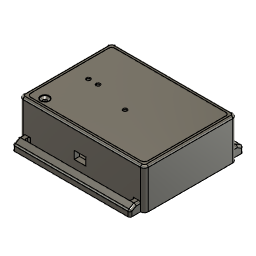
V5.0 Open-Source (Autodesk Fusion 360 design; units mm, degrees)
Autodesk Fusion 360 part; units mm, degrees
sketch "Top" plane through (0, 0, 0) normal (0, 1, 0) x (1, 0, 0)
  line L0 (35, -26.2) -> (48.95, -26.2) construction
  arc A0 (63, -48) -> (65, -46) centre (63, -46) ccw
  line L1 (63, -44) -> (63, -2)
  line L2 (38.05, -45.263) -> (25.05, -45.263)
  circle A1 centre (35, -26.2) radius 1.75
  line L3 (61.65, -14) -> (63, -14)
  line L4 (50.95, -35.25) -> (33, -35.25)
  line L5 (65, -2) -> (0, -2) construction
  circle A2 centre (35, -26.2) radius 1.4
  line L6 (39.475, -32.2956) -> (39.475, -27.2956)
  circle A3 centre (48.95, -26.2) radius 1.75
  line L7 (41.975, -26.2) -> (41.975, -27.2956) construction
  circle A4 centre (59.92, -22.92) radius 0.9 construction
  line L8 (58.127, -46) -> (58.127, -20.5)
  line L9 (25.05, -38.863) -> (38.05, -38.863) construction
  line L10 (30.3, -22) -> (33, -22)
  line L11 (2, 0) -> (63, 0)
  line L12 (2, -48) -> (63, -48)
  line L13 (39.55, -38.863) -> (39.55, -46) construction
  line L14 (3.35, -14) -> (2, -14)
  line L15 (29.5, -20.5) -> (29.5, -46) construction
  line L16 (2, -22) -> (30.3, -22) construction
  line L17 (63, -2) -> (2, -2)
  line L18 (63, -48) -> (63, 0) construction
  line L19 (61, -46) -> (4, -46)
  circle A5 centre (59.92, -43.58) radius 0.9 construction
  line L20 (25.05, -45.263) -> (25.05, -46)
  line L21 (50.95, -22) -> (58.127, -22)
  line L22 (38.05, -45.263) -> (38.05, -46)
  line L23 (38.05, -38.863) -> (39.55, -38.863) construction
  line L24 (33, -35.25) -> (33, -22)
  arc A6 (61, -46) -> (63, -44) centre (61, -44) ccw
  line L25 (2, -22) -> (0, -22) construction
  line L26 (2, -39.4) -> (30.3, -39.4)
  line L27 (30.3, -22) -> (30.3, -39.4)
  line L28 (2, -35.05) -> (25.085, -35.05)
  line L29 (39.475, -27.2956) -> (44.475, -27.2956)
  line L30 (44.475, -32.2956) -> (39.475, -32.2956)
  line L31 (2, -26.35) -> (25.085, -26.35)
  arc A7 (2, -44) -> (4, -46) centre (4, -44) ccw
  line L32 (33, -22) -> (50.95, -22)
  line L33 (65, -2) -> (65, -46)
  line L34 (0, -46) -> (0, -2)
  arc A8 (0, -46) -> (2, -48) centre (2, -46) ccw
  line L35 (38.05, -38.863) -> (38.05, -45.263) construction
  line L36 (25.085, -26.35) -> (25.085, -35.05)
  line L37 (6.88, -36.96) -> (6.88, -22) construction
  line L38 (25.05, -45.263) -> (25.05, -38.863) construction
  line L39 (23.55, -39.4) -> (23.55, -46)
  line L40 (0, -36.96) -> (6.88, -36.96) construction
  line L41 (2, -2) -> (2, -44)
  line L42 (8.127, -20.5) -> (8.127, -22)
  arc A9 (2, 0) -> (0, -2) centre (2, -2) ccw
  circle A10 centre (48.95, -26.2) radius 1.4
  line L43 (50.95, -22) -> (50.95, -35.25)
  line L44 (30.3, -39.4) -> (39.55, -39.4)
  arc A11 (65, -2) -> (63, 0) centre (63, -2) ccw
  line L45 (44.475, -27.2956) -> (44.475, -32.2956)
  line L46 (61.65, -17.5) -> (3.35, -17.5)
  line L47 (61.65, -14) -> (61.65, -2)
  line L48 (61.65, -17.5) -> (61.65, -14)
  line L49 (3.35, -14) -> (3.35, -2)
  line L50 (3.35, -17.5) -> (3.35, -14)
  line L51 (63, -19) -> (8.127, -19)
  line L52 (0, 0) -> (2, 0) construction
  line L53 (0, 0) -> (0, -2) construction
  line L54 (8.127, -20.5) -> (8.127, -19)
  circle A12 centre (8, -42.7) radius 2
  circle A13 centre (8, -42.7) radius 1
  line L55 (10.5, -46) -> (10.5, -39.4)
  line L56 (8.127, -22) -> (30.3, -22)
  line L57 (25.05, -39.4) -> (25.05, -45.263)
  line L58 (39.55, -39.4) -> (39.55, -46)
  line L59 (38.05, -39.4) -> (38.05, -45.263)
  line L60 (29.5, -20.5) -> (29.5, -22)
  line L61 (8.127, -20.5) -> (63, -20.5)
  line L62 (29.5, -22.6364) -> (36.034, -22.6364) construction
  line L63 (36.034, -22.6364) -> (36.9763, -20.5) construction
  line L64 (5.5, -39.4) -> (5.5, -46)
  line L65 (5.5, -45.2) -> (10.5, -45.2)
  line L66 (10.5, -40.2) -> (5.5, -40.2)
  line L67 (36.2744, -22) -> (36.936, -20.5)
  point P0 (0, -48)
  point P1 (65, 0)
  dimension "d1" = 65
  dimension "d2" = 48
  dimension "d3" = 2
  dimension "d9" = 2
  dimension "d10" = 2
  dimension "d11" = 33.5
  dimension "d12" = 4.873
  dimension "d14" = 13.25
  dimension "d15" = 17.95
  dimension "d16" = 3.5
  dimension "d17" = 2
  dimension "d18" = 28.3
  dimension "d19" = 28.3
  dimension "d20" = 17.4
  dimension "d22" = 6.88
  dimension "d23" = 14.96
  dimension "d24" = 2
  dimension "d26" = 6.4
  dimension "d27" = 13
  dimension "d28" = 0.737
  dimension "d29" = 23.05
  dimension "d30" = 1.8
  dimension "d31" = 1.8
  dimension "d32" = 2.42
  dimension "d33" = 3.08
  dimension "d34" = 3.08
  dimension "d36" = 3.5
  dimension "d37" = 3.5
  dimension "d38" = 2
  dimension "d39" = 2
  dimension "d40" = 4.2
  dimension "d41" = 4.2
  dimension "d42" = 90
  dimension "d44" = 5
  dimension "d45" = 5
  dimension "d46" = 90
  dimension "d47" = 2.8
  dimension "d48" = 2.8
  dimension "d49" = 1.5
  dimension "d50" = 1.5
  dimension "d51" = 4.35
  dimension "d129" = 2
  dimension "d133" = 2.9544
  dimension "d134" = 4.35
  dimension "d135" = 5.215
  dimension "d139" = 0.537
  dimension "d140" = 1.35
  dimension "d141" = 1.35
  dimension "d142" = 15.5
  dimension "d143" = 1.5
  dimension "d146" = 2
  dimension "d147" = 50
  dimension "d148" = 12
  dimension "d149" = 12
  dimension "d163" = 4
  dimension "d164" = 3.3
  dimension "d165" = 6
  dimension "d166" = 2
  dimension "d167" = 2.5
  dimension "d208" = 25.5
  dimension "d266" = 6.534
  dimension "d267" = 113.8
  dimension "d268" = 2.335
  dimension "d397" = 2.5
  dimension "d398" = 2.5
  dimension "d399" = 2.5
  dimension "d421" = 7.436
  constraint vertical L33
  constraint coincident L52.start L53.start
  constraint coincident L5.start L33
  constraint coincident L5.end L34
  constraint perpendicular L5 L34
  constraint coincident L1.end L18
  constraint coincident L1.end L5
  constraint coincident L17.end L5
  constraint coincident L3.end L18
  constraint perpendicular L3 L18
  constraint perpendicular L12 L33
  constraint coincident A0.start L12
  constraint perpendicular L11 L33
  constraint coincident L18.end L11
  constraint coincident L52.start L34
  constraint coincident L52.start L11
  constraint tangent L34 A9
  constraint tangent L11 A9
  constraint coincident P0 L34
  constraint coincident P0 L12
  constraint tangent L34 A8
  constraint tangent L12 A8
  constraint equal A8 A9
  constraint tangent A0 L33
  constraint tangent A0 L12
  constraint equal A0 A9
  constraint coincident P1 L33
  constraint coincident P1 L11
  constraint tangent L33 A11
  constraint tangent L11 A11
  constraint equal A9 A11
  constraint coincident L15.end L19
  constraint perpendicular L15 L19
  constraint coincident L8.start L19
  constraint horizontal L32
  constraint vertical L43
  constraint horizontal L4
  constraint vertical L24
  constraint tangent A7 L41
  constraint tangent L19 A7
  constraint tangent L19 A6
  constraint tangent L1 A6
  constraint equal A6 A7
  constraint coincident L26.start L41
  constraint perpendicular L26 L41
  constraint coincident L40.start L34
  constraint perpendicular L34 L40
  constraint coincident L37.end L16
  constraint perpendicular L16 L37
  constraint coincident L25.end L34
  constraint perpendicular L25 L34
  constraint horizontal L9
  constraint vertical L35
  constraint horizontal L2
  constraint vertical L38
  constraint coincident L42.end L16
  constraint perpendicular L16 L42
  constraint parallel L10 L32
  constraint coincident L21.end L8
  constraint perpendicular L8 L21
  constraint horizontal L29
  constraint vertical L45
  constraint horizontal L30
  constraint vertical L6
  constraint coincident L0.start A1.centre
  constraint coincident L0.end A3.centre
  constraint midpoint L7.start L0
  constraint midpoint L7.end L29
  constraint concentric A1 A2
  constraint concentric A3 A10
  constraint coincident L22.end L19
  constraint perpendicular L19 L22
  constraint coincident L20.end L19
  constraint perpendicular L19 L20
  constraint perpendicular L20 L23
  constraint coincident L13.end L19
  constraint perpendicular L13 L19
  constraint coincident L39.start L26
  constraint coincident L39.end L19
  constraint perpendicular L19 L39
  constraint coincident L44.end L13
  constraint perpendicular L13 L44
  constraint coincident L14.end L41
  constraint coincident L31.start L41
  constraint perpendicular L31 L41
  constraint coincident L28.start L41
  constraint perpendicular L28 L37
  constraint perpendicular L28 L36
  constraint coincident L17 L47.end
  constraint perpendicular L3 L47
  constraint perpendicular L3 L48
  constraint coincident L17 L49.end
  constraint perpendicular L14 L49
  constraint perpendicular L14 L50
  constraint coincident L1 L51.start
  constraint perpendicular L41 L51
  constraint tangent A9 L52
  constraint concentric A12 A13
  constraint coincident L19 L55.start
  constraint coincident L26 L55.end
  constraint perpendicular L26 L55
  constraint coincident L26 L57.start
  constraint coincident L38 L57.start
  constraint coincident L35 L59.start
  constraint coincident L44 L59.start
  constraint coincident L16 L60.end
  constraint coincident L1 L61.end
  constraint coincident L8.end L61
  constraint coincident L15.start L61
  constraint perpendicular L1 L61
  constraint perpendicular L54 L61
  constraint perpendicular L60 L61
  constraint coincident L15 L62.start
  constraint perpendicular L24 L62
  constraint coincident L61 L63.end
  constraint coincident L26 L64.start
  constraint coincident L19 L64.end
  constraint perpendicular L19 L64
  constraint coincident L64 L65.start
  constraint coincident L55 L65.end
  constraint perpendicular L55 L65
  constraint coincident L55 L66.start
  constraint coincident L64 L66.end
  constraint perpendicular L64 L66
  constraint coincident L32 L67.start
  constraint coincident L61 L67.end
  constraint parallel L63 L67
  measures "d1" distance of P1 L52.start
  measures "d2" distance of P0 L52.start
  measures "d3" distance of L18 L33
  measures "d9" radius of A9
  measures "d10" distance of L11 L17
  measures "d11" distance of L1 L15
  measures "d12" distance of L1 L8
  measures "d14" distance of L4 L32
  measures "d15" distance of L24 L43
  measures "d16" distance of L15 L24
  measures "d17" radius of A7
  measures "d18" distance of L26.start L26.end
  measures "d19" distance of L10.start L16.start
  measures "d20" distance of L16 L26
  measures "d22" distance of L37.start L40.start
  measures "d23" distance of L37.start L37.end
  measures "d24" distance of L34 L41
  measures "d26" distance of L2.end L9.start
  measures "d27" distance of L35 L38
  measures "d28" distance of L2 L19
  measures "d29" distance of L38 L41
  measures "d30" diameter of A5
  measures "d31" diameter of A4
  measures "d32" distance of A5.centre L19
  measures "d33" distance of A5.centre L1
  measures "d34" distance of A4.centre L18
  measures "d36" diameter of A1
  measures "d37" diameter of A3
  measures "d38" distance of L0.end L43
  measures "d39" distance of L0.start L24
  measures "d40" distance of L0.start L32
  measures "d41" distance of L0.end L32
  measures "d42" angle of L10 L27
  measures "d44" distance of L30.start L29.end
  measures "d45" distance of L6 L45
  measures "d46" angle of L0 L7
  measures "d47" diameter of A2
  measures "d48" diameter of A10
  measures "d49" distance of L9.end L13.start
  measures "d50" distance of L38 L39
  measures "d51" distance of L26 L28
  measures "d129" distance of L12 L19
  measures "d133" distance of L4 L30
  measures "d134" distance of L16 L31
  measures "d135" distance of L27 L36
  measures "d139" distance of L9 L26
  measures "d140" distance of L1 L47
  measures "d141" distance of L41 L49
  measures "d142" distance of L17 L46
  measures "d143" distance of L46 L51
  measures "d146" distance of L11.start L52.start
  measures "d147" distance of L8 L42
  measures "d148" distance of L14 L17
  measures "d149" distance of L3 L17
  measures "d163" diameter of A12
  measures "d164" distance of L19 A12.centre
  measures "d165" distance of L41 A12.centre
  measures "d166" diameter of A13
  measures "d167" distance of A12.centre L55
  measures "d208" distance of L19 L61
  measures "d266" distance of L62.start L62.end
  measures "d267" angle of L61 L63
  measures "d268" distance of L62.end L63.end
  measures "d397" distance of A12.centre L64
  measures "d398" distance of A12.centre L66
  measures "d399" distance of A12.centre L65
  measures "d421" distance of L15 L67.end
sketch "TP4056+JST" plane through (0, 0, 0) normal (1, 0, 0) x (0, 0, -1)
  line L0 (-22, 4.5) -> (-39.4, 4.5) construction
  line L1 (-26.4, 5.78) -> (-26.4, 5.86)
  arc A0 (-33.87, 8.205) -> (-35.87, 6.205) centre (-33.87, 6.205) ccw
  line L2 (-25.53, 5.435) -> (-25.53, 6.205)
  arc A1 (-35.87, 5.435) -> (-33.87, 3.435) centre (-33.87, 5.435) ccw
  arc A2 (-35, 5.78) -> (-33.65, 4.43) centre (-33.65, 5.78) ccw
  line L3 (-22, 3) -> (-22, 4.5) construction
  line L4 (-27.75, 7.21) -> (-33.65, 7.21)
  arc A3 (-27.75, 4.43) -> (-26.4, 5.78) centre (-27.75, 5.78) ccw
  arc A4 (-27.53, 3.435) -> (-25.53, 5.435) centre (-27.53, 5.435) ccw
  line L5 (-39.4, 4.5) -> (-39.4, 3) construction
  arc A5 (-25.53, 6.205) -> (-27.53, 8.205) centre (-27.53, 6.205) ccw
  line L6 (-33.87, 3.435) -> (-27.53, 3.435)
  line L7 (-35.87, 5.435) -> (-37.96, 5.435)
  line L8 (-37.96, 5.435) -> (-37.96, 8.435)
  line L9 (-35, 5.86) -> (-35, 5.78)
  line L10 (-33.65, 4.43) -> (-27.75, 4.43)
  line L11 (-30.7, 3) -> (-30.7, 7.21) construction
  line L12 (-25.53, 5.435) -> (-23.44, 5.435)
  line L13 (-27.53, 8.205) -> (-33.87, 8.205)
  arc A6 (-33.65, 7.21) -> (-35, 5.86) centre (-33.65, 5.86) ccw
  line L14 (-35.87, 6.205) -> (-35.87, 5.435)
  arc A7 (-26.4, 5.86) -> (-27.75, 7.21) centre (-27.75, 5.86) ccw
  line L15 (-23.44, 5.435) -> (-23.44, 8.435)
  line L16 (-39.4, 3) -> (-22, 3) construction
  line L17 (0, 0) -> (-48, 0)
  line L18 (-48, 0) -> (-48, 21)
  line L19 (-48, 21) -> (0, 21)
  line L20 (0, 21) -> (0, 0)
  line L21 (-25.44, 10.435) -> (-35.96, 10.435)
  line L22 (-44, 6) -> (-44, 9)
  line L23 (-43, 5) -> (-40, 5)
  line L24 (-39, 6) -> (-39, 9)
  line L25 (-40, 10) -> (-43, 10)
  arc A8 (-39, 9) -> (-40, 10) centre (-40, 9) ccw
  arc A9 (-43, 10) -> (-44, 9) centre (-43, 9) ccw
  arc A10 (-44, 6) -> (-43, 5) centre (-43, 6) ccw
  arc A11 (-40, 5) -> (-39, 6) centre (-40, 6) ccw
  line L26 (-37.96, 5.435) -> (-37.96, 3)
  line L27 (-23.44, 5.435) -> (-23.44, 3)
  line L28 (-25.53, 5.435) -> (-26.4448, 5.435)
  line L29 (-35.87, 5.435) -> (-34.9552, 5.435)
  line L30 (-23.44, 3) -> (-23.44, 1.5)
  line L31 (-23.44, 1.5) -> (-37.96, 1.5)
  line L32 (-37.96, 1.5) -> (-37.96, 3)
  arc A12 (-23.44, 8.435) -> (-25.44, 10.435) centre (-25.44, 8.435) ccw
  arc A13 (-35.96, 10.435) -> (-37.96, 8.435) centre (-35.96, 8.435) ccw
  point P0 (-26.4, 7.21)
  point P1 (-26.4, 4.43)
  point P2 (-35, 7.21)
  point P3 (-35.87, 8.205)
  point P4 (-25.53, 8.205)
  point P5 (-25.53, 3.435)
  point P6 (-23.44, 10.435)
  point P7 (-44, 5)
  dimension "d58" = 1.5
  dimension "d59" = 17.4
  dimension "d62" = 8.6
  dimension "d63" = 2.78
  dimension "d64" = 1.43
  dimension "d65" = 90
  dimension "d66" = 1.35
  dimension "d67" = 10.34
  dimension "d68" = 4.77
  dimension "d69" = 5.17
  dimension "d70" = 0.995
  dimension "d71" = 2
  dimension "d76" = 2.09
  dimension "d150" = 48
  dimension "d151" = 21
  dimension "d153" = 3.435
  dimension "d155" = 0.87
  dimension "d206" = 30.7
  dimension "d330" = 2.09
  dimension "d341" = 4
  dimension "d342" = 5
  dimension "d343" = 5
  dimension "d344" = 5
  dimension "d345" = 1
  dimension "d422" = 1.5
  dimension "d430" = 2
  dimension "d431" = 5
  constraint horizontal L0
  constraint vertical L5
  constraint horizontal L16
  constraint vertical L3
  constraint horizontal L4
  constraint vertical L9
  constraint horizontal L10
  constraint vertical L1
  constraint midpoint L11.start L16
  constraint coincident L11.end L4
  constraint coincident P0 L4
  constraint coincident P0 L1
  constraint tangent L4 A7
  constraint tangent L1 A7
  constraint coincident P2 L4
  constraint coincident P2 L9
  constraint tangent L4 A6
  constraint tangent L9 A6
  constraint equal A6 A7
  constraint tangent A2 L9
  constraint tangent A2 L10
  constraint equal A2 A7
  constraint coincident P1 L10
  constraint coincident P1 L1
  constraint tangent A3 L10
  constraint tangent L1 A3
  constraint equal A3 A7
  constraint horizontal L13
  constraint vertical L14
  constraint horizontal L6
  constraint vertical L2
  constraint coincident P4 L13
  constraint coincident P4 L2
  constraint tangent A5 L13
  constraint tangent L2 A5
  constraint coincident P3 L13
  constraint coincident P3 L14
  constraint tangent A0 L13
  constraint tangent A0 L14
  constraint equal A0 A5
  constraint tangent A1 L14
  constraint tangent A1 L6
  constraint equal A1 A5
  constraint coincident P5 L6
  constraint coincident P5 L2
  constraint tangent A4 L6
  constraint tangent L2 A4
  constraint equal A4 A5
  constraint perpendicular L2 L12
  constraint horizontal L17
  constraint vertical L18
  constraint horizontal L19
  constraint vertical L20
  constraint coincident L17.start L20.end
  constraint perpendicular L7 L8
  constraint horizontal L21
  constraint perpendicular L15 L21
  constraint vertical L22
  constraint perpendicular L22 L23
  constraint perpendicular L23 L24
  constraint perpendicular L24 L25
  constraint tangent L24 A8
  constraint tangent L25 A8
  constraint tangent L22 A9
  constraint tangent L25 A9
  constraint equal A8 A9
  constraint coincident P7 L22
  constraint coincident P7 L23
  constraint tangent L22 A10
  constraint tangent L23 A10
  constraint equal A8 A10
  constraint tangent L23 A11
  constraint tangent L24 A11
  constraint equal A8 A11
  constraint perpendicular L16 L26
  constraint coincident L16 L27.end
  constraint perpendicular L16 L27
  constraint coincident A3 L28.end
  constraint perpendicular L2 L28
  constraint coincident A2 L29.end
  constraint perpendicular L14 L29
  constraint perpendicular L16 L30
  constraint perpendicular L26 L31
  constraint perpendicular L16 L32
  constraint coincident P6 L15
  constraint tangent L21 A12
  constraint tangent L15 A12
  constraint tangent L8 A13
  constraint tangent L21 A13
  constraint equal A12 A13
  measures "d58" distance of L0 L16
  measures "d59" distance of L5.end L3.start
  measures "d62" distance of P0 P2
  measures "d63" distance of P0 P1
  measures "d64" distance of L10 L16
  measures "d65" angle of L11 L16
  measures "d66" radius of A7
  measures "d67" distance of P3 P4
  measures "d68" distance of P4 P5
  measures "d69" distance of L2 L11
  measures "d70" distance of L4 L13
  measures "d71" radius of A5
  measures "d76" distance of L2.start L12.end
  measures "d150" distance of L17.start L17.end
  measures "d151" distance of L17.start L19.end
  measures "d153" distance of L6 L17
  measures "d155" distance of L1 L2
  measures "d206" distance of L11 L20
  measures "d330" distance of L8 L14
  measures "d341" distance of L18 L22
  measures "d342" distance of L17 P7
  measures "d343" distance of L22 L24
  measures "d344" distance of L23 L25
  measures "d345" radius of A8
  measures "d422" distance of L17 L31
  measures "d430" radius of A12
  measures "d431" distance of L7 L21
ref_plane "WorkPlane2" through (0, 19, 0) normal (0, 1, 0) x (0, 0, 1)
sketch "Lid" plane through (0, 19, 0) normal (0, 1, 0) x (1, 0, 0)
  line L0 (0, 0) -> (65, 0) construction
  line L1 (65, 0) -> (65, -48) construction
  line L2 (65, -48) -> (0, -48) construction
  line L3 (0, -48) -> (0, 0) construction
  line L4 (62.95, -3.55) -> (62.95, -43.95)
  line L5 (60.95, -45.95) -> (4.05, -45.95)
  line L6 (2.05, -43.95) -> (2.05, -3.55)
  line L7 (3.55, -2.05) -> (61.45, -2.05)
  arc A0 (2.05, -43.95) -> (4.05, -45.95) centre (4.05, -43.95) ccw
  arc A1 (60.95, -45.95) -> (62.95, -43.95) centre (60.95, -43.95) ccw
  line L8 (2.05, -39.4) -> (30.35, -39.4) construction
  line L9 (30.35, -39.4) -> (30.35, -22) construction
  line L10 (30.35, -22) -> (2.05, -22) construction
  line L11 (28.35, -39.4) -> (28.35, -22) construction
  line L12 (62.95, -20.5) -> (36.953, -20.5) construction
  line L13 (36.953, -20.5) -> (36.1423, -22.3382) construction
  line L14 (35.6848, -22.6364) -> (29.9767, -22.6364) construction
  arc A2 (35.6848, -22.6364) -> (36.1423, -22.3382) centre (35.6848, -22.1364) ccw construction
  line L15 (29.4767, -23.1364) -> (29.4767, -45.95) construction
  arc A3 (29.9767, -22.6364) -> (29.4767, -23.1364) centre (29.9767, -23.1364) ccw construction
  line L16 (32.4767, -37.82) -> (29.4767, -37.82)
  line L17 (32.4767, -37.82) -> (32.4767, -39.82)
  line L18 (32.4767, -39.82) -> (29.4767, -39.82)
  line L19 (29.4767, -39.82) -> (29.4767, -37.82)
  line L20 (32.4767, -37.82) -> (32.4767, -28.68)
  line L21 (26.8767, -28.2) -> (29.2767, -28.2)
  line L22 (29.2767, -28.2) -> (29.2767, -33.2)
  line L23 (29.2767, -33.2) -> (26.8767, -33.2)
  line L24 (26.8767, -33.2) -> (26.8767, -28.2)
  line L25 (32.4767, -28.68) -> (29.4767, -28.68)
  line L26 (32.4767, -26.68) -> (29.4767, -26.68)
  line L27 (28.3767, -33.2) -> (28.3767, -28.2)
  line L28 (29.2767, -33.2) -> (29.4767, -33.2)
  line L29 (29.2767, -28.2) -> (29.4767, -28.2)
  line L30 (29.4767, -26.68) -> (29.4767, -28.2)
  line L31 (29.4767, -33.2) -> (29.4767, -37.82)
  line L32 (29.4767, -28.68) -> (29.4767, -28.2)
  circle A4 centre (34.026, -27.053) radius 0.75
  line L33 (32.4767, -28.68) -> (32.4767, -26.68)
  circle A5 centre (10.65, -22.7) radius 0.75
  circle A6 centre (15.65, -22.7) radius 0.75
  circle A7 centre (8, -42.7) radius 2.25
  line L34 (11.3, -45.95) -> (11.3, -39.4)
  line L35 (11.3, -39.4) -> (2.05, -39.4)
  circle A8 centre (8, -42.7) radius 1
  arc A9 (3.55, -2.05) -> (2.05, -3.55) centre (3.55, -3.55) ccw
  arc A10 (62.95, -3.55) -> (61.45, -2.05) centre (61.45, -3.55) ccw
  line L36 (60.95, -22.5) -> (59.95, -22.5)
  line L37 (58.95, -42.95) -> (58.95, -23.5)
  line L38 (58.163, -45.95) -> (58.163, -20.5) construction
  line L39 (61.95, -23.5) -> (61.95, -42.95)
  line L40 (60.95, -43.95) -> (59.95, -43.95)
  arc A11 (61.95, -23.5) -> (60.95, -22.5) centre (60.95, -23.5) ccw
  arc A12 (59.95, -22.5) -> (58.95, -23.5) centre (59.95, -23.5) ccw
  arc A13 (58.95, -42.95) -> (59.95, -43.95) centre (59.95, -42.95) ccw
  arc A14 (60.95, -43.95) -> (61.95, -42.95) centre (60.95, -42.95) ccw
  point P0 (36.0107, -22.6364)
  point P1 (29.4767, -22.6364)
  dimension "d98" = 65
  dimension "d99" = 48
  dimension "d101" = 2
  dimension "d102" = 6.55
  dimension "d103" = 28.3
  dimension "d104" = 17.4
  dimension "d105" = 2
  dimension "d106" = 25.45
  dimension "d109" = 25.997
  dimension "d110" = 113.8
  dimension "d112" = 6.534
  dimension "d113" = 2.335
  dimension "d114" = 0.5
  dimension "d115" = 0.5
  dimension "d116" = 8.13
  dimension "d117" = 2
  dimension "d121" = 6.2
  dimension "d122" = 5
  dimension "d123" = 2
  dimension "d124" = 9.14
  dimension "d125" = 0.2
  dimension "d126" = 2.4
  dimension "d127" = 1.5
  dimension "d128" = 3
  dimension "d171" = 1.5
  dimension "d172" = 18.897
  dimension "d173" = 28.924
  dimension "d174" = 1.5
  dimension "d175" = 1.5
  dimension "d176" = 8.6
  dimension "d177" = 23.25
  dimension "d178" = 5
  dimension "d179" = 4.5
  dimension "d181" = 3.25
  dimension "d182" = 5.95
  dimension "d183" = 3.3
  dimension "d231" = 2
  dimension "d316" = 1.5
  dimension "d434" = 4.787
  dimension "d436" = 3
  dimension "d437" = 1
  dimension "d438" = 1
  dimension "d439" = 2
  dimension "d440" = 2
  constraint horizontal L0
  constraint vertical L1
  constraint horizontal L2
  constraint vertical L3
  constraint coincident L0.start L3.end
  constraint tangent L5 A0
  constraint tangent L6 A0
  constraint tangent L4 A1
  constraint tangent L5 A1
  constraint equal A0 A1
  constraint coincident L6 L8.start
  constraint perpendicular L6 L8
  constraint perpendicular L8 L9
  constraint coincident L6 L10.end
  constraint perpendicular L6 L10
  constraint coincident L8 L11.start
  constraint coincident L10 L11.end
  constraint perpendicular L10 L11
  constraint coincident L4 L12.start
  constraint perpendicular L4 L12
  constraint horizontal L14
  constraint coincident P0 L13
  constraint coincident P0 L14
  constraint tangent L13 A2
  constraint tangent L14 A2
  constraint coincident L5 L15.end
  constraint perpendicular L5 L15
  constraint coincident P1 L14
  constraint coincident P1 L15
  constraint tangent L14 A3
  constraint tangent L15 A3
  constraint perpendicular L15 L16
  constraint perpendicular L16 L17
  constraint perpendicular L15 L18
  constraint perpendicular L16 L19
  constraint perpendicular L16 L20
  constraint perpendicular L11 L21
  constraint perpendicular L21 L22
  constraint perpendicular L22 L23
  constraint perpendicular L21 L24
  constraint coincident L15 L25.end
  constraint perpendicular L15 L25
  constraint coincident L15 L26.end
  constraint perpendicular L15 L26
  constraint coincident L23 L27.start
  constraint coincident L21 L27.end
  constraint perpendicular L21 L27
  constraint coincident L15 L28.end
  constraint perpendicular L15 L28
  constraint coincident L15 L29.end
  constraint perpendicular L15 L29
  constraint perpendicular L16 L31
  constraint perpendicular L26 L33
  constraint horizontal A5.centre A6.centre
  constraint coincident L5 L34.start
  constraint coincident L8 L34.end
  constraint perpendicular L8 L34
  constraint concentric A7 A8
  constraint tangent L6 A9
  constraint tangent L7 A9
  constraint tangent L4 A10
  constraint tangent L7 A10
  constraint equal A9 A10
  constraint coincident L5 L38.start
  constraint coincident L12 L38.end
  constraint perpendicular L12 L38
  constraint perpendicular L37 L40
  constraint perpendicular L36 L37
  constraint perpendicular L36 L39
  constraint parallel L4 L39
  constraint tangent L36 A11
  constraint tangent L39 A11
  constraint tangent L36 A12
  constraint tangent L37 A12
  constraint equal A11 A12
  constraint tangent L37 A13
  constraint tangent L40 A13
  constraint equal A11 A13
  constraint tangent L39 A14
  constraint tangent L40 A14
  constraint equal A11 A14
  measures "d98" distance of L0.start L0.end
  measures "d99" distance of L0.start L2.end
  measures "d101" radius of A0
  measures "d102" distance of L5 L8
  measures "d103" distance of L8.start L8.end
  measures "d104" distance of L8.end L9.end
  measures "d105" distance of L9 L11
  measures "d106" distance of L5 L12
  measures "d109" distance of L4 L12.end
  measures "d110" angle of L12 L13
  measures "d112" distance of P0 P1
  measures "d113" distance of L12.end P0
  measures "d114" radius of A2
  measures "d115" radius of A3
  measures "d116" distance of L5 L16
  measures "d117" distance of L16.start L17.end
  measures "d121" distance of L8 L23
  measures "d122" distance of L21 L23
  measures "d123" distance of L25 L26
  measures "d124" distance of L16 L25
  measures "d125" distance of L15 L22
  measures "d126" distance of L21.start L21.end
  measures "d127" distance of L24 L27
  measures "d128" distance of L15 L20
  measures "d171" diameter of A4
  measures "d172" distance of L5 A4.centre
  measures "d173" distance of L4 A4.centre
  measures "d174" diameter of A5
  measures "d175" diameter of A6
  measures "d176" distance of L6 A5.centre
  measures "d177" distance of L5 A5.centre
  measures "d178" distance of A5.centre A6.centre
  measures "d179" diameter of A7
  measures "d181" distance of L5 A7.centre
  measures "d182" distance of L6 A7.centre
  measures "d183" distance of A7.centre L34
  measures "d231" diameter of A8
  measures "d316" radius of A9
  measures "d434" distance of L4 L38
  measures "d436" distance of L37 L39
  measures "d437" radius of A11
  measures "d438" distance of L4 L39
  measures "d439" distance of L5 L40
  measures "d440" distance of L12 L36
extrude "Extrude10" add sketch "Top" along normal blind 1.5 contours L1 L3 L14 L26 L27 L28 L31 L36 L41 L42 L46 L48 L50 L51 L54 L56 | L4 L24 L32 L43 makes body 1 at (28.5617, 0, 32.15) makes body 2 at (48.0814, 0, 31.8302)
extrude "Extrude11" add sketch "Top" along normal blind 3 contours L17 L46 L47 L48 L49 L50 | L28 L31 L36 L41 | A1 | L6 L29 L30 L45 | A3 bodies 1 2
extrude "Extrude12" add sketch "Top" along normal blind 5 contours L4 L8 L10 L19 L21 L24 L27 L43 L44 L58 | L42 L56 L60 L61 | L2 L26 L44 L57 L59 | L19 L26 L39 L55 bodies 1 2
extrude "Extrude13" add sketch "Top" along normal blind 11.8 contours L1 L8 L19 A6 L61 | L8 L21 L32 L61 L67 | L10 L32 L56 L60 L61 L67 | L19 L22 L44 L58 L59 | L2 L19 L20 L22 | L19 L20 L26 L39 L57 | A2 | A10 bodies 1
extrude "Extrude16" add sketch "Top" along normal blind 21 contours A0 L11 L12 L33 L34 A8 A9 A11 bodies 1
extrude "Extrude20" add sketch "Lid" against normal blind 17.5 separate body contours L21 L22 L23 L27 makes body 3
extrude "Extrude21" add sketch "Lid" against normal blind 14.5 contours L21 L23 L24 L27 bodies 3
extrude "Extrude22" add sketch "Lid" against normal blind 3 contours L16 L20 L22 L25 L28 L29 L31 L32 bodies 3
extrude "Extrude23" add sketch "Lid" against normal blind 6.2 contours L16 L17 L18 L19 | L25 L26 L30 L32 L33 bodies 3
chamfer "Chamfer2" distance 0.5 angle 45 2 edges at (33.6947, 11.8, 26.7063) (47.6447, 11.8, 26.7063) on bodies 1
extrude "Extrude30" add sketch "Top" along normal blind 19 contours L10 L32 L56 L60 L61 L67 bodies 1
fillet "Fillet3" radius 1 8 edges at (32.5, 21, 48) (64.4142, 21, 47.4142) (65, 21, 24) (64.4142, 21, 0.5858) (32.5, 21, 0) (0.5858, 21, 0.5858) (0, 21, 24) (0.5858, 21, 47.4142) on bodies 1
sketch "Strap Loop" plane through (0, 0, 0) normal (-1, 0, 0) x (0, 0, 1)
  line L0 (46, 20) -> (2, 20)
  line L1 (2, 20) -> (2, 0)
  line L2 (2, 0) -> (46, 0)
  line L3 (46, 0) -> (46, 20)
  line L4 (0, 0) -> (48, 0)
  line L5 (48, 0) -> (48, 21)
  line L6 (48, 21) -> (0, 21)
  line L7 (0, 21) -> (0, 0)
  line L8 (48, 0) -> (50.5, 0)
  line L9 (50.5, 0) -> (53.5, 0)
  line L10 (53.5, 0) -> (53.5, 3)
  line L11 (50.5, 0) -> (50.5, 4.7321)
  line L12 (53.5, 3) -> (50.5, 4.7321)
  line L13 (50.5, 4.7321) -> (48, 4.7321)
  line L14 (24, 0) -> (24, 21) construction
  line L15 (0, 0) -> (-2.5, 0)
  line L16 (-5.5, 0) -> (-5.5, 3)
  line L17 (-5.5, 3) -> (-2.5, 4.7321)
  line L18 (-2.5, 0) -> (-5.5, 0)
  line L19 (-2.5, 0) -> (-2.5, 4.7321)
  line L20 (-2.5, 4.7321) -> (0, 4.7321)
  dimension "d283" = 48
  dimension "d284" = 21
  dimension "d285" = 2.5
  dimension "d286" = 3
  dimension "d287" = 3
  dimension "d289" = 120
  constraint horizontal L4
  constraint vertical L5
  constraint horizontal L6
  constraint vertical L7
  constraint coincident L4.start L7.end
  constraint perpendicular L5 L8
  constraint parallel L8 L9
  constraint perpendicular L9 L10
  constraint perpendicular L8 L11
  constraint coincident L5 L13.end
  constraint perpendicular L5 L13
  constraint midpoint L4 L14.start
  constraint midpoint L6 L14.end
  constraint coincident L4.end L5.start
  constraint symmetric L4.end L14 L4.start
  constraint symmetric L8.end L14 L15.end
  constraint symmetric L9.end L14 L16.start
  constraint symmetric L10.end L14 L16.end
  constraint symmetric L11.end L14 L17.end
  constraint symmetric L13.end L14 L20.end
  measures "d283" distance of L4.start L4.end
  measures "d284" distance of L4.start L6.end
  measures "d285" distance of L4.end L8.end
  measures "d286" distance of L8.end L9.end
  measures "d287" distance of L9.end L10.end
  measures "d289" angle of L10 L12
extrude "Extrude31" add sketch "Strap Loop" along normal blind -2 and the other way blind 63 separate body contours L9 L10 L11 L12 | L16 L17 L18 L19 makes body 4 at (42.6667, 1.5774, 50.5) makes body 5 at (22.3333, 1.5774, -2.5)
extrude "Extrude32" add sketch "Strap Loop" along normal blind -2 and the other way blind 5 contours L5 L8 L11 L13 | L7 L15 L19 L20 | L9 L10 L11 L12 | L16 L17 L18 L19 bodies 4 1 5
extrude "Extrude33" add sketch "Strap Loop" along normal blind -60 and the other way blind 63 contours L5 L8 L11 L13 | L7 L15 L19 L20 | L9 L10 L11 L12 | L16 L17 L18 L19 bodies 4
extrude "Extrude34" add sketch "Lid" against normal blind 6.2 separate body contours L36 L37 L39 L40 A11 A12 A13 A14 makes body 6
extrude "Extrude35" add sketch "Lid" along normal blind 2 contours L4 L5 L6 L7 A1 L34 L35 A9 A10 | L5 L6 A0 L34 L35 | L16 L17 L18 L19 | L16 L20 L22 L25 L28 L29 L31 L32 | L25 L26 L30 L32 L33 | L21 L22 L23 L27 | L21 L23 L24 L27 | L36 L37 L39 L40 A11 A12 A13 A14 bodies 3 6
extrude "Extrude37" add sketch "Top" along normal blind 5 contours L19 L55 L64 L65 | L19 L26 A7 L41 L64 | L55 L64 L65 L66 | L26 L55 L64 L66 bodies 4
extrude "Extrude38" add sketch "Top" along normal blind 19 contours L1 L51 L54 L61 | L1 L3 L17 L47 | L14 L17 L41 L49 | L55 L64 L65 L66 | A12 bodies 4
fillet "Fillet20" radius 2 4 edges at (5.5, 12, 40.2) (10.5, 12, 40.2) (10.5, 12, 45.2) (5.5, 12, 45.2) on bodies 4
extrude "Extrude39" add sketch "Top" along normal blind 12 contours A13 bodies 4
fillet "Fillet12" radius 1.5 2 edges at (63, 20, 2) (2, 20, 2) on bodies 4
extrude "Extrude40" cut sketch "TP4056+JST" along normal blind 2 contours L1 A2 L4 A3 L9 L10 A6 A7 | L1 A0 L2 A2 L4 A3 A5 L9 L13 A6 L14 A7 L28 L29 | A1 A2 A3 A4 L6 L10 L28 L29 | L22 L23 L24 L25 A8 A9 A10 A11 bodies 4
extrude "Extrude41" add sketch "TP4056+JST" along normal blind 5 and the other way blind -1.25 contours L1 A0 L2 A2 L4 A3 A5 L9 L13 A6 L14 A7 L28 L29 | A0 L2 A5 L7 L8 L12 L13 L14 L15 L21 A12 A13 bodies 4
extrude "Extrude46" add sketch "TP4056+JST" along normal blind 2.5 and the other way blind -1.25 contours A1 A2 A3 A4 L6 L10 L28 L29 | A1 A4 L6 L7 L12 L26 L27 L30 L31 L32 bodies 4
chamfer "Chamfer4" distance 1 angle 45 3 edges at (5, 7.21, 30.7) (5, 6.8146, 34.6046) (5, 6.8146, 26.7954) on bodies 4
fillet "Fillet13" radius 0.8 8 edges at (60, 2.366, 0) (60, 2.366, -2.5) (5, 2.366, 0) (5, 2.366, -2.5) (5, 2.366, 48) (5, 2.366, 50.5) (60, 2.366, 50.5) (60, 2.366, 48) on bodies 4
fillet "Fillet14" radius 1 4 edges at (63, 1.5, 53.5) (2, 1.5, 53.5) (2, 1.5, -5.5) (63, 1.5, -5.5) on bodies 4
fillet "Fillet15" radius 1 14 edges at (2, 4.1547, -3.5) (2.2929, 3.1691, -5.2071) (32.5, 3, -5.5) (62.7071, 3.1691, -5.2071) (63, 4.1547, -3.5) (2, 4.1547, 51.5) (2.2929, 3.1691, 53.2071) (32.5, 3, 53.5) (62.7071, 3.1691, 53.2071) (63, 4.1547, 51.5) (63, 4.7321, 49.25) (2, 4.7321, 49.25) (2, 4.7321, -1.25) (63, 4.7321, -1.25) on bodies 4
extrude "Extrude42" add sketch "Lid" along normal blind 1.8 contours A7 bodies 3
chamfer "Chamfer5" distance 1 angle 45 1 edges at (7.0677, 20.8, 42.3384) on bodies 3
fillet "Fillet16" radius 0.3 3 edges at (14.9508, 21, 22.4288) (9.9508, 21, 22.4288) (33.3268, 21, 26.7818) on bodies 3
fillet "Fillet17" radius 0.5 8 edges at (0, 5.82, 25.53) (0, 7.6192, 26.1158) (0, 8.205, 30.7) (0, 7.6192, 35.2842) (0, 5.82, 35.87) (0, 4.0208, 35.2842) (0, 3.435, 30.7) (0, 4.0208, 26.1158) on bodies 4
ref_plane "WorkPlane3" through (0, 0, 48) normal (0, 0, 1) x (1, 0, 0)
sketch "Switch" plane through (0, 0, 48) normal (0, 0, 1) x (1, 0, 0)
  line L0 (0, 0) -> (65, 0)
  line L1 (65, 0) -> (65, 21)
  line L2 (65, 21) -> (0, 21)
  line L3 (0, 21) -> (0, 0)
  line L4 (23.55, 11.8) -> (23.55, 5)
  line L5 (25.05, 11.8) -> (25.05, 5)
  line L6 (0, 5) -> (65, 5) construction
  line L7 (23.55, 11.8) -> (25.05, 11.8)
  line L8 (25.05, 11.8) -> (38.05, 11.8)
  line L9 (38.05, 11.8) -> (38.05, 5)
  line L10 (38.05, 11.8) -> (39.55, 11.8)
  line L11 (39.55, 11.8) -> (39.55, 5)
  line L12 (28.55, 10.435) -> (34.55, 10.435)
  line L13 (34.55, 10.435) -> (34.55, 6.365)
  line L14 (34.55, 6.365) -> (28.55, 6.365)
  line L15 (28.55, 6.365) -> (28.55, 10.435)
  line L16 (25.05, 11.8) -> (25.05, 19)
  line L17 (25.05, 19) -> (23.55, 19)
  line L18 (23.55, 19) -> (23.55, 11.8)
  line L19 (25.05, 19) -> (29.45, 19)
  line L20 (29.45, 19) -> (29.45, 11.8)
  dimension "d372" = 65
  dimension "d373" = 21
  dimension "d374" = 23.55
  dimension "d375" = 1.5
  dimension "d376" = 5
  dimension "d377" = 6.8
  dimension "d378" = 13
  dimension "d379" = 1.5
  dimension "d380" = 1.365
  dimension "d381" = 1.365
  dimension "d382" = 3.5
  dimension "d383" = 3.5
  dimension "d384" = 19
  dimension "d386" = 35.55
  constraint horizontal L0
  constraint vertical L1
  constraint horizontal L2
  constraint vertical L3
  constraint coincident L0.start L3.end
  constraint vertical L4
  constraint vertical L5
  constraint coincident L3 L6.start
  constraint coincident L1 L6.end
  constraint perpendicular L1 L6
  constraint coincident L4.end L6
  constraint coincident L5.end L6
  constraint perpendicular L4 L7
  constraint perpendicular L5 L8
  constraint coincident L6 L9.end
  constraint perpendicular L6 L9
  constraint perpendicular L9 L10
  constraint coincident L6 L11.end
  constraint perpendicular L6 L11
  constraint horizontal L12
  constraint vertical L13
  constraint horizontal L14
  constraint vertical L15
  constraint perpendicular L7 L16
  constraint perpendicular L16 L17
  constraint perpendicular L17 L18
  constraint coincident L16 L17.start
  constraint perpendicular L16 L19
  constraint coincident L8 L20.end
  constraint perpendicular L8 L20
  constraint coincident L16.end L17.start
  measures "d372" distance of L0.start L0.end
  measures "d373" distance of L0.start L2.end
  measures "d374" distance of L3 L4
  measures "d375" distance of L4 L5
  measures "d376" distance of L0 L6
  measures "d377" distance of L6 L7
  measures "d378" distance of L5.start L8.end
  measures "d379" distance of L9 L11
  measures "d380" distance of L6 L14
  measures "d381" distance of L8 L12
  measures "d382" distance of L5 L15
  measures "d383" distance of L9 L13
  measures "d384" distance of L0 L17
  measures "d386" distance of L1 L20
extrude "Extrude43" cut sketch "Switch" against normal blind 2.737 contours L12 L13 L14 L15 bodies 4
extrude "Extrude44" add sketch "Switch" against normal blind 8.6 contours L7 L16 L17 L18 bodies 4
extrude "Extrude45" add sketch "Switch" against normal blind 2.737 contours L8 L16 L19 L20 bodies 4
fillet "Fillet18" radius 2 6 edges at (25.085, 2.25, 35.05) (25.085, 2.25, 26.35) (39.475, 2.25, 32.2956) (44.475, 2.25, 32.2956) (44.475, 2.25, 27.2956) (39.475, 2.25, 27.2956) on bodies 1 2 4
fillet "Fillet19" radius 2 2 edges at (3.35, 2.25, 17.5) (61.65, 2.25, 17.5) on bodies 4
fillet "Fillet21" radius 0.75 2 edges at (8.127, 10.25, 19) (8.127, 12, 20.5) on bodies 4
fillet "Fillet22" radius 1 1 edges at (8.127, 3.25, 22) on bodies 4
fillet "Fillet23" radius 0.75 1 edges at (29.5, 12, 22) on bodies 4
fillet "Fillet24" radius 0.75 1 edges at (29.5, 12, 20.5) on bodies 4
fillet "Fillet28" radius 0.75 4 edges at (39.55, 8.4, 39.4) (38.05, 8.4, 39.4) (25.05, 12, 39.4) (23.55, 12, 39.4) on bodies 1 4
fillet "Fillet29" radius 2 4 edges at (23.55, 12, 46) (39.55, 8.4, 46) (58.127, 8.4, 46) (58.127, 8.4, 22) on bodies 4
chamfer "Chamfer8" distance 0.5 angle 45 3 edges at (2.5, 4.43, 30.7) (2.5, 4.7104, 26.9264) (2.5, 4.7104, 34.4736) on bodies 4
fillet "Fillet30" radius 1 4 edges at (32.4767, 15.9, 39.82) (29.4767, 15.9, 39.82) (32.4767, 15.9, 26.68) (29.4767, 15.9, 26.68) on bodies 3
fillet "Fillet31" radius 1 2 edges at (26.8767, 11.75, 28.2) (26.8767, 11.75, 33.2) on bodies 3
fillet "Fillet32" radius 0.4 4 edges at (28.3767, 3, 28.2) (28.3767, 3, 33.2) (29.2767, 8.75, 28.2) (29.2767, 8.75, 33.2) on bodies 3
fillet "Fillet33" radius 1 4 edges at (32.4767, 14.4, 37.82) (32.4767, 14.4, 28.68) (29.4767, 14.4, 37.82) (29.4767, 14.4, 28.68) on bodies 3
fillet "Fillet34" radius 0.65 6 edges at (61.65, 2.25, 14) (61.65, 11, 14) (63, 10.25, 14) (3.35, 11, 14) (3.35, 2.25, 14) (2, 10.25, 14) on bodies 4
fillet "Fillet35" radius 1 2 edges at (63, 10.25, 19) (63, 15.4, 20.5) on bodies 4
fillet "Fillet36" radius 0.75 1 edges at (36.2744, 15.4, 22) on bodies 4
named bodies: "Case Body", "V5.0 Lid", "V5.0 Case Body"
